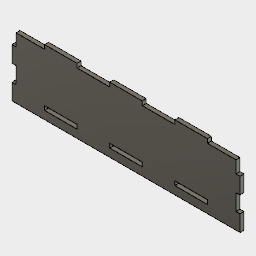
base_frontside v1 (Autodesk Fusion 360 design; units mm, degrees)
Autodesk Fusion 360 part; units mm, degrees
sketch "スケッチ1" plane through (0, 0, 0) normal (0, 0, 1) x (1, 0, 0)
  line L0 (227.26, -118.9783) -> (227.26, -121.4783)
  line L1 (127.2604, -118.9783) -> (147.2604, -118.9783)
  line L2 (227.26, -121.4783) -> (207.2598, -121.4783)
  line L3 (147.2604, -118.9783) -> (147.2604, -121.4783)
  line L4 (207.2598, -121.4783) -> (207.2598, -118.9783)
  line L5 (187.2604, -121.4783) -> (167.2602, -121.4783)
  line L6 (207.2598, -118.9783) -> (227.26, -118.9783)
  line L7 (187.2604, -118.9783) -> (187.2604, -121.4783)
  line L8 (167.2602, -121.4783) -> (167.2602, -118.9783)
  line L9 (167.2602, -118.9783) -> (187.2604, -118.9783)
  line L10 (244.7608, -88.9781) -> (227.2604, -88.9781)
  line L11 (227.2604, -88.9781) -> (227.2604, -86.478)
  line L12 (227.2604, -86.478) -> (207.2605, -86.478)
  line L13 (207.2605, -86.478) -> (207.2605, -88.9781)
  line L14 (207.2605, -88.9781) -> (187.2604, -88.9781)
  line L15 (187.2604, -88.9781) -> (187.2604, -86.478)
  line L16 (187.2604, -86.478) -> (167.2604, -86.478)
  line L17 (167.2604, -86.478) -> (167.2604, -88.9781)
  line L18 (167.2604, -88.9781) -> (147.2604, -88.9781)
  line L19 (147.2604, -88.9781) -> (147.2604, -86.478)
  line L20 (147.2604, -86.478) -> (127.2604, -86.478)
  line L21 (127.2604, -86.478) -> (127.2604, -88.9781)
  line L22 (127.2604, -88.9781) -> (109.7603, -88.9781)
  line L23 (109.7603, -88.9781) -> (109.7603, -96.4781)
  line L24 (109.7603, -96.4781) -> (107.2604, -96.4781)
  line L25 (107.2604, -96.4781) -> (107.2604, -106.4782)
  line L26 (107.2604, -106.4782) -> (109.7603, -106.4782)
  line L27 (109.7603, -106.4782) -> (109.7603, -116.4782)
  line L28 (109.7603, -116.4782) -> (107.2604, -116.4782)
  line L29 (107.2604, -116.4782) -> (107.2604, -126.4783)
  line L30 (107.2604, -126.4783) -> (109.7603, -126.4783)
  line L31 (109.7603, -126.4783) -> (244.7608, -126.4783)
  line L32 (244.7608, -126.4783) -> (247.2605, -126.4783)
  line L33 (247.2605, -126.4783) -> (247.2605, -116.4782)
  line L34 (247.2605, -116.4782) -> (244.7608, -116.4782)
  line L35 (244.7608, -116.4782) -> (244.7608, -106.4782)
  line L36 (244.7608, -106.4782) -> (247.2605, -106.4782)
  line L37 (247.2605, -106.4782) -> (247.2605, -96.4781)
  line L38 (247.2605, -96.4781) -> (244.7608, -96.4781)
  line L39 (244.7608, -96.4781) -> (244.7608, -88.9781)
  line L40 (147.2604, -121.4783) -> (127.2604, -121.4783)
  line L41 (127.2604, -121.4783) -> (127.2604, -118.9783)
extrude "押し出し1" add sketch "スケッチ1" along normal blind 2.5
